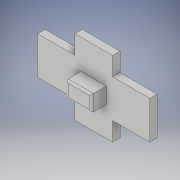
# Autodesk Inventor part: palm_plate
Saved by Autodesk Inventor 2019 (Build 230136000, 136)
## iProperties
Created: 2024-08-27
Part Number: palm_plate
Material: Generisch
Document SubType Name: Modeling
Designer: nic
Density: 1 g/cm^3
Appearance: Vorgabe
Author: nic
Autodesk Inventor part; units mm, degrees
ref_plane "YZ Plane" through (0, 0, 0) normal (1, 0, 0) x (0, 1, 0)
ref_plane "XZ Plane" through (0, 0, 0) normal (0, 1, 0) x (-1, 0, 0)
ref_plane "XY Plane" through (0, 0, 0) normal (0, 0, 1) x (1, 0, 0)
sketch "Skizze2" plane through (0, 0, 0) normal (0, 0, 1) x (1, 0, 0)
  line L0 (47.429, 1.628) -> (41.9536, 1.5965) projected
  line L1 (47.4645, -1.7719) -> (41.9641, -1.8346) projected
  line L2 (41.9168, 1.5642) -> (41.9437, -0.1365) projected
  line L3 (47.466, 0.6928) -> (47.4706, 0.1306) projected
  line L4 (48.1143, -2.2865) -> (41.3143, -2.2865)
  line L5 (41.3143, -2.2865) -> (41.3143, 2.0135)
  line L6 (41.3143, 2.0135) -> (48.1143, 2.0135)
  line L7 (48.1143, 2.0135) -> (48.1143, -2.2865)
  line L8 (48.1143, -2.2865) -> (41.3143, 2.0135) construction
  line L9 (41.3143, -2.2865) -> (48.1143, 2.0135) construction
  point P0 (0, 0)
  point P1 (44.7143, -0.1365)
  dimension "d0" = 6.8
  dimension "d1" = 4.3
  constraints: 12 end point, 2 midpoint, 2 parallel, 1 horizontal, 1 perpendicular
  measures "d0" distance of L5.end L6.end
  measures "d1" distance of L4.end L5.end
extrude "Extrusion1" add sketch "Skizze2" against normal blind 6
sketch "Skizze4" plane through (0, 0, -6) normal (0, 0, -1) x (-1, 0, 0)
  line L0 (-48.1143, -2.2865) -> (-41.3143, -2.2865) construction
  line L1 (-41.3143, 2.0135) -> (-48.1143, 2.0135) construction
  line L2 (-41.3143, -2.2865) -> (-41.3143, 2.0135) construction
  line L3 (-48.1143, 2.0135) -> (-48.1143, -2.2865) construction
  line L4 (-49.8143, -10.2365) -> (-39.6143, -10.2365)
  line L5 (-39.6143, -10.2365) -> (-39.6143, 9.9635)
  line L6 (-39.6143, 9.9635) -> (-49.8143, 9.9635)
  line L7 (-49.8143, -10.2365) -> (-39.6143, 9.9635) construction
  line L8 (-39.6143, -10.2365) -> (-49.8143, 9.9635) construction
  line L9 (-59.8143, -5.2365) -> (-59.8143, 4.9635)
  line L10 (-29.6143, -5.2365) -> (-59.8143, 4.9635) construction
  line L11 (-59.8143, -5.2365) -> (-29.6143, 4.9635) construction
  line L12 (-41.3143, -5.2365) -> (-42.1391, -5.2365)
  line L13 (-49.8143, -5.2365) -> (-59.8143, -5.2365)
  line L14 (-59.8143, 4.9635) -> (-49.8143, 4.9635)
  line L15 (-42.1391, 4.9635) -> (-41.3143, 4.9635)
  line L16 (-49.8143, 9.9635) -> (-49.8143, 4.9635)
  line L17 (-49.8143, -5.2365) -> (-49.8143, -10.2365)
  point P0 (0, 0)
  point P1 (-44.7143, -0.1365)
  point P2 (-44.7143, -0.1365)
  constraints: 28 end point, 7 parallel, 5 midpoint, 4 point on line, 3 horizontal, 3 perpendicular
extrude "Extrusion2" add sketch "Skizze4" along normal blind 2
fillet "Rundung1" radius 1 4 edges at (44.7143, 2.0135, 0) (41.3143, -0.1365, 0) (48.1143, -0.1365, 0) (44.7143, -2.2865, 0)
sketch "Skizze5" plane through (0, 0, 0) normal (0, 0, 1) x (1, 0, 0)
  line L0 (49.8143, -10.2365) -> (39.6143, -10.2365) projected
  line L1 (49.8143, -5.2365) -> (49.8143, -10.2365) projected
  line L2 (59.8143, -5.2365) -> (49.8143, -5.2365) projected
  line L3 (59.8143, 4.9635) -> (59.8143, -5.2365) projected
  line L4 (49.8143, 4.9635) -> (59.8143, 4.9635) projected
  line L5 (49.8143, 9.9635) -> (49.8143, 4.9635) projected
  line L6 (39.6143, 9.9635) -> (49.8143, 9.9635) projected
  line L7 (39.6143, -10.2365) -> (39.6143, 9.9635) projected
  line L8 (48.1143, 2.0135) -> (48.1143, -2.2865) projected
  line L9 (48.1143, -2.2865) -> (41.3143, -2.2865) projected
  line L10 (41.3143, -2.2865) -> (41.3143, 2.0135) projected
  line L11 (41.3143, 2.0135) -> (48.1143, 2.0135) projected
  point P0 (0, 0)
extrude "Extrusion3" cut sketch "Skizze5" against normal blind 2 contours L8 L9 L10 L11
fillet "Rundung2" radius 0.5 4 edges at (44.7143, 2.0135, -2) (41.3143, -0.1365, -2) (44.7143, -2.2865, -2) (48.1143, -0.1365, -2)
sketch "Skizze6" plane through (0, 0, -8) normal (0, 0, -1) x (-1, 0, 0)
  line L0 (-49.8143, -10.2365) -> (-39.6143, -10.2365) projected
  line L1 (-39.6143, -10.2365) -> (-39.6143, 9.9635) projected
  line L2 (-39.6143, 9.9635) -> (-49.8143, 9.9635) projected
  line L3 (-49.8143, 9.9635) -> (-49.8143, 4.9635) projected
  line L4 (-49.8143, 4.9635) -> (-59.8143, 4.9635) projected
  line L5 (-59.8143, 4.9635) -> (-59.8143, -5.2365) projected
  line L6 (-59.8143, -5.2365) -> (-49.8143, -5.2365) projected
  line L7 (-49.8143, -5.2365) -> (-49.8143, -10.2365) projected
  line L8 (-39.6143, -10.2365) -> (-39.6143, 9.9635) projected
  line L9 (-39.6143, 4.9635) -> (-29.6143, 4.9635)
  line L10 (-29.6143, 4.9635) -> (-29.6143, -5.2365)
  line L11 (-29.6143, -5.2365) -> (-39.6143, -5.2365)
  line L12 (-39.6143, -5.2365) -> (-39.6143, 4.9635)
  point P0 (0, 0)
  dimension "d14" = 10
  constraints: 8 end point, 2 parallel, 1 horizontal, 1 perpendicular, 1 point on line
  measures "d14" distance of L10.end L11.end
extrude "Extrusion4" add sketch "Skizze6" against normal up to surface (2 mm away) contours L1 L9 L10 L11
